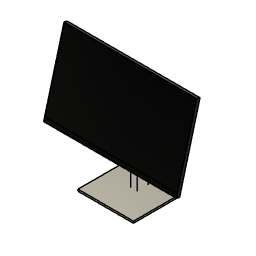
Desk-V1 (Autodesk Fusion 360 archive; units mm, degrees)
design "Screen"
Autodesk Fusion 360 part; units mm, degrees
sketch "Skizze1" plane through (0, 0, 0) normal (0, 0, 1) x (1, 0, 0)
  line L0 (-25, 15) -> (230, 15)
  line L1 (230, 15) -> (230, -190)
  line L2 (230, -190) -> (-25, -190)
  line L3 (-25, -190) -> (-25, 15)
  line L4 (87.5, -10) -> (117.5, -10)
  line L5 (117.5, -10) -> (117.5, -60)
  line L6 (117.5, -60) -> (87.5, -60)
  line L7 (87.5, -60) -> (87.5, -10)
  dimension "d1" = 255
  dimension "d2" = 205
  dimension "d3" = 30
  dimension "d4" = 50
  dimension "d5" = 25
  dimension "d6" = 112.5
  constraint horizontal L0
  constraint vertical L1
  constraint horizontal L2
  constraint vertical L3
  constraint horizontal L4
  constraint vertical L5
  constraint horizontal L6
  constraint vertical L7
  measures "d1" distance of L0.start L0.end
  measures "d2" distance of L0.start L2.end
  measures "d3" distance of L4.start L4.end
  measures "d4" distance of L4.start L6.end
  measures "d5" distance of L0 L4
  measures "d6" distance of L1 L5
extrude "Extrusion1" add sketch "Skizze1" along normal blind 8 contours L0 L1 L2 L3 | L4 L5 L6 L7 makes body 1
sketch "Skizze2" plane through (0, -190, 0) normal (0, -1, 0) x (1, 0, 0)
  line L0 (-25, 0) -> (230, 0)
  line L1 (230, 0) -> (230, 8)
  line L2 (230, 8) -> (-25, 8)
  line L3 (-25, 8) -> (-25, 0)
  line L4 (-202.5, 540) -> (407.5, 540)
  line L5 (407.5, 540) -> (407.5, 178)
  line L6 (407.5, 178) -> (-202.5, 178)
  line L7 (-202.5, 178) -> (-202.5, 540)
  dimension "d10" = 610
  dimension "d11" = 362
  dimension "d12" = 170
  dimension "d13" = 177.5
  dimension "d14" = 177.5
  constraint horizontal L4
  constraint vertical L5
  constraint horizontal L6
  constraint vertical L7
  measures "d10" distance of L4.start L4.end
  measures "d11" distance of L4.end L5.end
  measures "d12" distance of L2 L6
  measures "d13" horizontal distance of L2.end L6.end
  measures "d14" distance of L1.end L5
extrude "Extrusion2" add sketch "Skizze2" along normal blind 15 separate body contours L4 L5 L6 L7 makes body 2
move_body "Verschieben1" bodies 2 to x (1, 0, 0) y (0, 1, 0) z (0, 0, 1) at (0, 15, 0)
move_body "Verschieben2" bodies 2 to x (1, 0, 0) y (0, 0.965926, -0.258819) z (0, 0.258819, 0.965926) at (0, -52.5439, -43.1104)
move_body "Verschieben3" bodies 2 to x (1, 0, 0) y (0, 1, 0) z (0, 0, 1) at (0, 20, 0)
move_body "Verschieben4" bodies 2 to x (1, 0, 0) y (0, 1, 0) z (0, 0, 1) at (0, 30, 0)
extrude "Extrusion3" add sketch "Skizze1" along normal blind 388 separate body contours L4 L5 L6 L7 makes body 3
move_body "Verschieben5" bodies 2 to x (1, 0, 0) y (0, 1, 0) z (0, 0, 1) at (0, -30, 0)
sketch "Skizze3" plane through (0, -60, 0) normal (0, -1, 0) x (1, 0, 0)
  line L0 (87.5, 0) -> (117.5, 0)
  line L1 (117.5, 0) -> (117.5, 388)
  line L2 (117.5, 388) -> (87.5, 388)
  line L3 (87.5, 388) -> (87.5, 0)
  line L4 (87.5, 388) -> (117.5, 388)
  line L5 (117.5, 388) -> (117.5, 348)
  line L6 (117.5, 348) -> (87.5, 348)
  line L7 (87.5, 348) -> (87.5, 388)
  dimension "d19" = 40
  constraint horizontal L4
  constraint vertical L5
  constraint horizontal L6
  constraint vertical L7
  constraint coincident L1 L5.end
  constraint coincident L2.end L3.start
  measures "d19" distance of L1.end L5.end
extrude "Extrusion4" add sketch "Skizze3" along normal blind 55 separate body contours L1 L2 L3 L4 L5 L6 L7 makes body 4
ref_plane "Arbeitsebene1" through (102.5, -108.6649, 348.9503) normal (0, 0.965926, -0.258819) x (-1, 0, 0)
split "Teilen1" by plane through (102.5, -108.6649, 348.9503) normal (0, 0.965926, -0.258819) bodies 4 makes body 5 at (117.5, -89.0403, 361.3333)
delete_body "Körper entfernen1" bodies 4
sketch "Skizze4" plane through (0, -203.1122, 54.4237) normal (0, -0.965926, 0.258819) x (1, 0, 0)
  line L0 (-202.5, 127.9356) -> (407.5, 127.9356)
  line L1 (407.5, 127.9356) -> (407.5, 489.9356)
  line L2 (407.5, 489.9356) -> (-202.5, 489.9356)
  line L3 (-202.5, 489.9356) -> (-202.5, 127.9356)
  line L4 (-200.5, 487.9356) -> (405.5, 487.9356)
  line L5 (405.5, 487.9356) -> (405.5, 145.9356)
  line L6 (405.5, 145.9356) -> (-200.5, 145.9356)
  line L7 (-200.5, 145.9356) -> (-200.5, 487.9356)
  dimension "d25" = 2
  dimension "d26" = 2
  dimension "d27" = 2
  dimension "d28" = 18
  constraint horizontal L4
  constraint vertical L5
  constraint horizontal L6
  constraint vertical L7
  measures "d25" distance of L1 L5
  measures "d26" distance of L3 L7
  measures "d27" distance of L2 L4
  measures "d28" distance of L0 L6
extrude "Extrusion6" cut sketch "Skizze4" against normal blind 0.01 contours L4 L5 L6 L7 bodies 2
equation "d17 = 380 mm + 8 mm"
named bodies: "baseplate", "screen", "stand", "stand-arm"

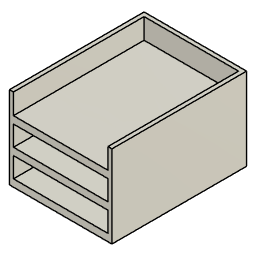
design "Ablagefach-A4"
Autodesk Fusion 360 part; units mm, degrees
sketch "Skizze1" plane through (0, 0, 0) normal (0, 0, 1) x (1, 0, 0)
  line L0 (-15, 30) -> (240, 30)
  line L1 (240, 30) -> (240, -305)
  line L2 (240, -305) -> (-15, -305)
  line L3 (-15, -305) -> (-15, 30)
  dimension "d1" = 255
  dimension "d2" = 335
  constraint horizontal L0
  constraint vertical L1
  constraint horizontal L2
  constraint vertical L3
  measures "d1" distance of L0.start L0.end
  measures "d2" distance of L0.start L2.end
extrude "Extrusion1" add sketch "Skizze1" along normal blind 205
sketch "Skizze2" plane through (0, -305, 0) normal (0, -1, 0) x (1, 0, 0)
  line L0 (-15, 0) -> (240, 0)
  line L1 (240, 0) -> (240, 205)
  line L2 (240, 205) -> (-15, 205)
  line L3 (-15, 205) -> (-15, 0)
sketch "Skizze3" plane through (0, -305, 0) normal (0, -1, 0) x (1, 0, 0)
  line L0 (-5, 205) -> (-15, 205)
  line L1 (-15, 205) -> (-15, 0)
  line L2 (-15, 0) -> (-5, 0)
  line L3 (-5, 0) -> (-5, 205)
  line L4 (230, 0) -> (240, 0)
  line L5 (240, 0) -> (240, 205)
  line L6 (240, 205) -> (230, 205)
  line L7 (230, 205) -> (230, 0)
  line L8 (-5, 0) -> (230, 0)
  line L9 (230, 0) -> (230, 18)
  line L10 (230, 18) -> (-5, 18)
  line L11 (-5, 18) -> (-5, 0)
  line L12 (-5, 68) -> (230, 68)
  line L13 (230, 68) -> (230, 86)
  line L14 (230, 86) -> (-5, 86)
  line L15 (-5, 86) -> (-5, 68)
  line L16 (-5, 154) -> (230, 154)
  line L17 (230, 154) -> (230, 136)
  line L18 (230, 136) -> (-5, 136)
  line L19 (-5, 136) -> (-5, 154)
  line L20 (240, 205) -> (-15, 205)
  dimension "d8" = 235
  dimension "d9" = 10
  dimension "d12" = 10
  dimension "d13" = 205
  dimension "d14" = 18
  dimension "d15" = 50
  dimension "d16" = 18
  dimension "d17" = 50
  dimension "d18" = 18
  dimension "d19" = 51
  constraint horizontal L0
  constraint vertical L1
  constraint horizontal L2
  constraint vertical L3
  constraint horizontal L4
  constraint vertical L5
  constraint horizontal L6
  constraint vertical L7
  constraint horizontal L8
  constraint vertical L9
  constraint horizontal L10
  constraint vertical L11
  constraint coincident L7 L9.end
  constraint horizontal L12
  constraint vertical L13
  constraint horizontal L14
  constraint vertical L15
  constraint coincident L7 L13.end
  constraint horizontal L16
  constraint vertical L17
  constraint horizontal L18
  constraint vertical L19
  constraint coincident L7 L17.end
  constraint coincident L3 L16.start
  measures "d8" distance of L3 L7
  measures "d9" distance of L4.start L4.end
  measures "d12" distance of L1.end L2.end
  measures "d13" distance of L4.start L6.end
  measures "d14" distance of L2.end L10.end
  measures "d15" distance of L10 L12
  measures "d16" distance of L12.start L14.end
  measures "d17" distance of L14 L18
  measures "d18" distance of L16 L18
  measures "d19" distance of L16 L20
extrude "Extrusion2" cut sketch "Skizze3" against normal blind 325 contours L3 L7 L16 L20 | L3 L7 L14 L18 | L3 L7 L10 L12

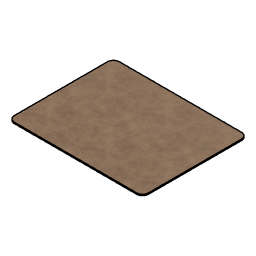
design "Mousepad"
Autodesk Fusion 360 part; units mm, degrees
sketch "Skizze1" plane through (0, 0, 0) normal (0, 0, 1) x (1, 0, 0)
  line L0 (-12.0523, 42.3584) -> (197.9477, 42.3584)
  line L1 (207.9477, 32.3584) -> (207.9477, -127.6416)
  line L2 (197.9477, -137.6416) -> (-12.0523, -137.6416)
  line L3 (-22.0523, -127.6416) -> (-22.0523, 32.3584)
  arc A0 (-12.0523, 42.3584) -> (-22.0523, 32.3584) centre (-12.0523, 32.3584) ccw
  arc A1 (207.9477, 32.3584) -> (197.9477, 42.3584) centre (197.9477, 32.3584) ccw
  arc A2 (197.9477, -137.6416) -> (207.9477, -127.6416) centre (197.9477, -127.6416) ccw
  arc A3 (-22.0523, -127.6416) -> (-12.0523, -137.6416) centre (-12.0523, -127.6416) ccw
  point P0 (-22.0523, 42.3584)
  point P1 (207.9477, 42.3584)
  point P2 (-22.0523, -137.6416)
  dimension "d1" = 230
  dimension "d2" = 180
  dimension "d3" = 10
  constraint horizontal L0
  constraint vertical L1
  constraint horizontal L2
  constraint vertical L3
  constraint coincident P0 L0
  constraint coincident P0 L3
  constraint tangent L0 A0
  constraint tangent L3 A0
  constraint coincident P1 L0
  constraint coincident P1 L1
  constraint tangent L0 A1
  constraint tangent L1 A1
  constraint equal A0 A1
  constraint tangent L1 A2
  constraint tangent L2 A2
  constraint equal A0 A2
  constraint coincident P2 L2
  constraint coincident P2 L3
  constraint tangent L2 A3
  constraint tangent L3 A3
  constraint equal A0 A3
  measures "d1" distance of P0 P1
  measures "d2" distance of P0 P2
  measures "d3" radius of A0
extrude "Extrusion1" add sketch "Skizze1" along normal blind 2
named bodies: "body"

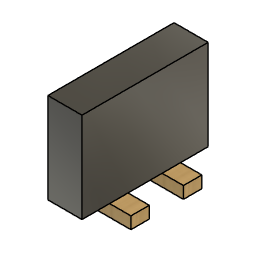
design "Computer"
Autodesk Fusion 360 part; units mm, degrees
sketch "Skizze1" plane through (0, 0, 0) normal (0, 0, 1) x (1, 0, 0)
  line L0 (-250, 20) -> (-25, 20)
  line L1 (-25, 20) -> (-25, -34)
  line L2 (-25, -34) -> (-250, -34)
  line L3 (-250, -34) -> (-250, 20)
  line L4 (-250, 20) -> (-25, 20)
  line L5 (-25, -34) -> (-250, -34)
  line L6 (-250, -34) -> (-250, 20)
  line L7 (-25, 20) -> (-25, -34)
  line L8 (-25, -188) -> (-250, -188)
  line L9 (-25, -134) -> (-25, -188)
  line L10 (-250, -188) -> (-250, -134)
  line L11 (-250, -134) -> (-25, -134)
  dimension "d3" = 225
  dimension "d4" = 54
  dimension "d5" = 225
  dimension "d6" = 54
  dimension "d9" = 225
  dimension "d10" = 54
  dimension "d11" = 100
  constraint horizontal L0
  constraint vertical L1
  constraint horizontal L2
  constraint vertical L3
  constraint horizontal L4
  constraint vertical L7
  constraint horizontal L5
  constraint vertical L6
  constraint horizontal L11
  constraint vertical L9
  constraint horizontal L8
  constraint vertical L10
  measures "d3" distance of L0.start L0.end
  measures "d4" distance of L0.start L2.end
  measures "d5" distance of L0.end L0.start
  measures "d6" distance of L0.start L2.end
  measures "d9" distance of L10.end L9.start
  measures "d10" distance of L10.end L8.end
  measures "d11" distance of L5 L11
extrude "Extrusion1" add sketch "Skizze1" along normal blind 35 makes body 1 at (-175, 2, 0) makes body 2 at (-100, -170, 0)
sketch "Skizze2" plane through (0, 0, 35) normal (0, 0, 1) x (-1, 0, 0)
  line L0 (25, -20) -> (250, -20)
  line L1 (250, -20) -> (250, 34)
  line L2 (250, 34) -> (25, 34)
  line L3 (25, 34) -> (25, -20)
  line L4 (187.5, -101) -> (87.5, -101)
  line L5 (87.5, -101) -> (87.5, 269)
  line L6 (87.5, 269) -> (187.5, 269)
  line L7 (187.5, 269) -> (187.5, -101)
  line L8 (25, 134) -> (25, 188)
  line L9 (250, 188) -> (250, 134)
  line L10 (25, 188) -> (250, 188)
  line L11 (250, -20) -> (25, -20)
  dimension "d14" = 100
  dimension "d15" = 370
  dimension "d18" = 81
  dimension "d19" = 81
  dimension "d20" = 62.5
  dimension "d21" = 62.5
  constraint horizontal L4
  constraint vertical L5
  constraint horizontal L6
  constraint vertical L7
  measures "d14" distance of L4.start L4.end
  measures "d15" distance of L4.start L6.end
  measures "d18" distance of L6 L10
  measures "d19" distance of L4 L11
  measures "d20" distance of L7 L9
  measures "d21" distance of L5 L8
extrude "Extrusion2" add sketch "Skizze2" along normal blind 265 separate body contours L0 L2 L5 L7 L11 | L0 L4 L5 L7 L11 | L2 L5 L7 L10 | L5 L6 L7 L10 makes body 3
named bodies: "Bodenabstand-2", "Bodenabstand-1", "PC"

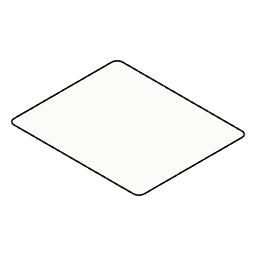
design "Deskpad"
Autodesk Fusion 360 part; units mm, degrees
sketch "Skizze1" plane through (0, 0, 0) normal (0, 0, 1) x (1, 0, 0)
  line L0 (125, 150) -> (1225, 150)
  line L1 (1275, 100) -> (1275, -800)
  line L2 (1225, -850) -> (125, -850)
  line L3 (75, -800) -> (75, 100)
  arc A0 (125, 150) -> (75, 100) centre (125, 100) ccw
  arc A1 (1275, 100) -> (1225, 150) centre (1225, 100) ccw
  arc A2 (1225, -850) -> (1275, -800) centre (1225, -800) ccw
  arc A3 (75, -800) -> (125, -850) centre (125, -800) ccw
  point P0 (75, 150)
  point P1 (1275, 150)
  point P2 (75, -850)
  dimension "d1" = 1200
  dimension "d2" = 1000
  dimension "d3" = 50
  dimension "d4" = 50
  constraint horizontal L0
  constraint vertical L1
  constraint horizontal L2
  constraint vertical L3
  constraint coincident P0 L0
  constraint coincident P0 L3
  constraint tangent L0 A0
  constraint tangent L3 A0
  constraint coincident P1 L0
  constraint coincident P1 L1
  constraint tangent L0 A1
  constraint tangent L1 A1
  constraint equal A0 A1
  constraint tangent L1 A2
  constraint tangent L2 A2
  constraint equal A0 A2
  constraint coincident P2 L2
  constraint coincident P2 L3
  constraint tangent L2 A3
  constraint tangent L3 A3
  measures "d1" distance of P0 P1
  measures "d2" distance of P0 P2
  measures "d3" radius of A0
  measures "d4" radius of A3
extrude "Extrusion1" add sketch "Skizze1" along normal blind 2
equation "d4 = d3"
named bodies: "body"

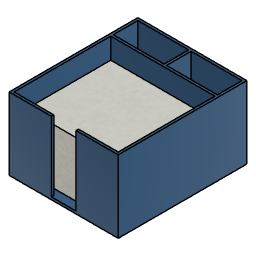
design "Paperholder"
Autodesk Fusion 360 part; units mm, degrees
sketch "Skizze1" plane through (0, 0, 0) normal (0, 0, 1) x (1, 0, 0)
  line L0 (-45, 50) -> (44, 50)
  line L1 (44, 50) -> (44, -55)
  line L2 (44, -55) -> (-45, -55)
  line L3 (-45, -55) -> (-45, 50)
  line L4 (-43, 48) -> (42, 48)
  line L5 (42, 48) -> (42, -53)
  line L6 (42, -53) -> (-43, -53)
  line L7 (-43, -53) -> (-43, 48)
  line L8 (-10.5, -53) -> (9.5, -53)
  line L9 (9.5, -53) -> (9.5, -55)
  line L10 (9.5, -55) -> (-10.5, -55)
  line L11 (-10.5, -55) -> (-10.5, -53)
  line L12 (-43, 27.9185) -> (42, 27.9185)
  line L13 (42, 27.9185) -> (42, 25.9185)
  line L14 (42, 25.9185) -> (-43, 25.9185)
  line L15 (-43, 25.9185) -> (-43, 27.9185)
  line L16 (-1.5, 48) -> (0.5, 48)
  line L17 (0.5, 48) -> (0.5, 27.9185)
  line L18 (0.5, 27.9185) -> (-1.5, 27.9185)
  line L19 (-1.5, 27.9185) -> (-1.5, 48)
  dimension "d1" = 89
  dimension "d2" = 105
  dimension "d3" = 2
  dimension "d4" = 2
  dimension "d5" = 2
  dimension "d6" = 2
  dimension "d7" = 20
  dimension "d8" = 34.5
  dimension "d9" = 34.5
  dimension "d10" = 2
  dimension "d11" = 2
  dimension "d12" = 41.5
  dimension "d13" = 85
  dimension "d14" = 41.5
  constraint horizontal L0
  constraint vertical L1
  constraint horizontal L2
  constraint vertical L3
  constraint horizontal L4
  constraint vertical L5
  constraint horizontal L6
  constraint vertical L7
  constraint horizontal L8
  constraint vertical L9
  constraint horizontal L10
  constraint vertical L11
  constraint coincident L2 L9.end
  constraint coincident L6 L8.start
  constraint horizontal L12
  constraint vertical L13
  constraint horizontal L14
  constraint vertical L15
  constraint coincident L5 L13.end
  constraint coincident L7 L12.start
  constraint horizontal L16
  constraint vertical L17
  constraint horizontal L18
  constraint vertical L19
  constraint coincident L12 L17.end
  constraint coincident L4 L16.start
  measures "d1" distance of L0.start L0.end
  measures "d2" distance of L0.start L2.end
  measures "d3" distance of L1 L5
  measures "d4" distance of L3 L7
  measures "d5" distance of L0 L4
  measures "d6" distance of L2 L6
  measures "d7" distance of L8.start L8.end
  measures "d8" distance of L3 L11
  measures "d9" distance of L1 L9
  measures "d10" distance of L16.start L16.end
  measures "d11" distance of L12 L14
  measures "d12" distance of L5 L17
  measures "d13" distance of L4.start L4.end
  measures "d14" distance of L7 L19
extrude "Extrusion1" add sketch "Skizze1" along normal blind 2 contours L5 L6 L7 L8 L14 | L4 L7 L12 L19 | L4 L5 L12 L17 makes body 1 at (13.6667, -26.6938, 0) makes body 2 at (28.1667, 34.6123, 0) makes body 3 at (-29.1667, 41.3062, 0)
extrude "Extrusion2" add sketch "Skizze1" along normal blind 59 contours L0 L1 L2 L3 L4 L5 L6 L7 L9 L11 L13 L15 L16 | L5 L7 L12 L13 L14 L15 L18 | L4 L12 L16 L17 L18 L19 bodies 1 2 3
extrude "Extrusion3" add 1 faces at (2.8333, -53, 0.6667) along direction (0, -1, 0) blind 2 on bodies 1 bodies 1
sketch "Skizze2" plane through (0, 0, 2) normal (0, 0, 1) x (-1, 0, 0)
  line L0 (-42, 53) -> (-42, -25.9185)
  line L1 (-42, -25.9185) -> (43, -25.9185)
  line L2 (43, -25.9185) -> (43, 53)
  line L3 (43, 53) -> (10.5, 53)
  line L4 (10.5, 53) -> (10.5, 55)
  line L5 (10.5, 55) -> (-9.5, 55)
  line L6 (-9.5, 55) -> (-9.5, 53)
  line L7 (-9.5, 53) -> (-42, 53)
  line L8 (38, -20.9185) -> (-37, -20.9185)
  line L9 (-37, -20.9185) -> (-37, 48)
  line L10 (-37, 48) -> (38, 48)
  line L11 (38, 48) -> (38, -20.9185)
  dimension "d21" = 5
  dimension "d22" = 5
  dimension "d23" = 5
  dimension "d24" = 5
  constraint horizontal L8
  constraint vertical L9
  constraint horizontal L10
  constraint vertical L11
  measures "d21" distance of L0 L9
  measures "d22" distance of L2 L11
  measures "d23" distance of L3 L10
  measures "d24" distance of L1 L8
extrude "Extrusion4" add sketch "Skizze2" along normal blind 45 separate body contours L8 L9 L10 L11 makes body 4
named bodies: "main", "sticky-notes"
